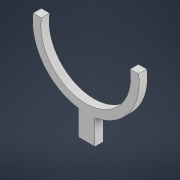
# Autodesk Inventor part: Clip_TestFitV1
Saved by Autodesk Inventor 2022 (Build 260153000, 153)
## iProperties
Created: 2023-05-05
Part Number: Clip_TestFitV1
Material: Generic
Document SubType Name: Modeling
Designer: User
Density: 1 g/cm^3
Appearance: Default
Author: User
Autodesk Inventor part; units mm, degrees
ref_plane "YZ Plane" through (0, 0, 0) normal (1, 0, 0) x (0, 1, 0)
ref_plane "XZ Plane" through (0, 0, 0) normal (0, 1, 0) x (-1, 0, 0)
ref_plane "XY Plane" through (0, 0, 0) normal (0, 0, 1) x (1, 0, 0)
sketch "Sketch1" plane through (0, 0, 0) normal (0, 0, 1) x (1, 0, 0)
  arc A0 (-27.1622, 4.2969) -> (27.1622, 4.2969) centre (0, 0) ccw
  line L0 (-27.1622, 4.2969) -> (-32.2159, 4.2969)
  line L1 (27.1622, 4.2969) -> (32.3878, 4.4173)
  line L2 (27.1622, 4.2969) -> (32.3878, 4.4173) construction
  line L3 (5.608, -32.5424) -> (5.608, -47.5424)
  line L4 (5.608, -47.5424) -> (-4.392, -47.5424)
  line L5 (-4.392, -47.5424) -> (-4.392, -32.5424)
  line L6 (-4.392, -32.5424) -> (-4.392, -32.203)
  line L7 (5.608, -32.5424) -> (5.608, -32.203)
  arc A1 (-32.2159, 4.2969) -> (-4.392, -32.203) centre (0, 0) ccw
  arc A2 (5.608, -32.203) -> (32.3878, 4.4173) centre (0, 0) ccw
  dimension "d0" = 55
  dimension "d5" = 10
  dimension "d6" = 15
  constraints: 16 end point, 6 point on circle, 3 centre point, 2 coincident, 1 parallel, 1 vertical
  measures "d0" diameter of A0
  measures "d5" distance of L3.end L4.end
  measures "d6" distance of L3.start L3.end
extrude "Extrusion1" add sketch "Sketch1" along normal blind 5
body "Solid1"
